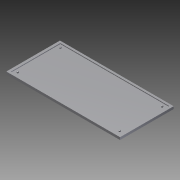
# Autodesk Inventor part: BoxCover
Saved by Autodesk Inventor 2012 SP2 (Build 160219200, 219)
## iProperties
Created: 2013-08-24
Part Number: BoxCover
Material: Default
Document SubType Name: Modeling
Designer: 1
Density: 1 g/cm^3
Author: 1
Autodesk Inventor part; units mm, degrees
ref_plane "YZ Plane" through (0, 0, 0) normal (1, 0, 0) x (0, 1, 0)
ref_plane "XZ Plane" through (0, 0, 0) normal (0, 1, 0) x (-1, 0, 0)
ref_plane "XY Plane" through (0, 0, 0) normal (0, 0, 1) x (1, 0, 0)
sketch "Sketch1" plane through (0, 0, 0) normal (0, 0, 1) x (1, 0, 0)
  line L0 (350, -225) -> (-350, -225) projected
  line L1 (-335, 210) -> (335, 210) projected
  line L2 (335, 210) -> (335, -210) projected
  line L3 (335, -210) -> (-335, -210) projected
  line L4 (-335, -210) -> (-335, 210) projected
  line L5 (350, -225) -> (-350, -225) projected
  line L6 (350, 225) -> (350, -225) projected
  line L7 (-350, 225) -> (350, 225) projected
  line L8 (-350, -225) -> (-350, 225) projected
  line L9 (350, -210) -> (-350, -210)
  line L10 (-350, -225) -> (350, -225)
  point P0 (0, 0)
  constraints: 4 end point, 2 point on line, 1 collinear, 1 perpendicular
extrude "Extrusion1" add sketch "Sketch1" along normal blind 330.2 contours L0 L8 L9 L3 L6
sketch "Sketch2" plane through (-350, -210, 0) normal (0, 1, 0) x (1, 0, 0)
  line L0 (0, -330.2) -> (700, -330.2) projected
  line L1 (700, 0) -> (700, -330.2) projected
  line L2 (700, 0) -> (0, 0) projected
  line L3 (0, 0) -> (0, -330.2) projected
  line L4 (15, 0) -> (685, 0) projected
  line L5 (15, 0) -> (15, -330.2) construction
  line L6 (685, 0) -> (685, -330.2) construction
  line L7 (0, -12.7) -> (700, -12.7) construction
  line L8 (0, -317.5) -> (700, -317.5) construction
  line L9 (15, -12.7) -> (685, -12.7) construction
  line L10 (685, -12.7) -> (685, -317.5) construction
  line L11 (685, -317.5) -> (15, -317.5) construction
  line L12 (15, -317.5) -> (15, -12.7) construction
  line L13 (15, -317.5) -> (685, -317.5)
  line L14 (685, -317.5) -> (685, -12.7)
  line L15 (685, -12.7) -> (15, -12.7)
  line L16 (15, -12.7) -> (15, -317.5)
  point P0 (350, 0)
  dimension "d2" = 12.7
  dimension "d3" = 12.7
  constraints: 24 end point, 10 point on line, 6 perpendicular, 4 parallel, 2 horizontal
  measures "d2" distance between parallel lines of L2 L7
  measures "d3" distance between parallel lines of L0 L8
extrude "Extrusion2" cut sketch "Sketch2" against normal blind 4.7625 contours L16 L15 L14 L13
sketch "Sketch3" plane through (-350, -214.7625, 0) normal (0, 1, 0) x (1, 0, 0)
  line L0 (685, -12.7) -> (15, -12.7) projected
  line L1 (15, -12.7) -> (15, -317.5) projected
  line L2 (15, -317.5) -> (685, -317.5) projected
  line L3 (685, -317.5) -> (685, -12.7) projected
  line L4 (36.7157, -34.4157) -> (663.2843, -34.4157) construction
  line L5 (663.2843, -34.4157) -> (663.2843, -295.7843) construction
  line L6 (663.2843, -295.7843) -> (36.7157, -295.7843) construction
  line L7 (36.7157, -295.7843) -> (36.7157, -34.4157) construction
  circle A0 centre (36.7157, -34.4157) radius 5.1916
  circle A1 centre (663.2843, -34.4157) radius 5.1916
  circle A2 centre (663.2843, -295.7843) radius 5.1916
  circle A3 centre (36.7157, -295.7843) radius 5.1916
  point P0 (350, 0)
  dimension "d6" = 21.7157
  dimension "d7" = 10.3831
  constraints: 8 end point, 4 centre point, 4 coincident, 3 equal radius, 3 other
  measures "d6" distance between parallel lines of L0 L4
  measures "d7" diameter of A0
extrude "Extrusion3" add sketch "Sketch3" along normal blind 7.62 contours A0 | A1 | A2 | A3
fillet "Fillet1" radius 3.175 4 edges at (308.0927, -207.1425, 34.4157) (308.0927, -207.1425, 295.7843) (-318.4758, -207.1425, 295.7843) (-318.4758, -207.1425, 34.4157)
body "Solid1"
